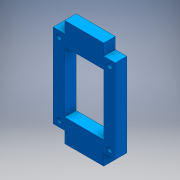
# Autodesk Inventor part: backFrame
Saved by Autodesk Inventor 2016 (Build 200138000, 138)
## iProperties
Created: 2016-06-05
Part Number: backFrame
Material: Generic
Document SubType Name: Modeling
Designer: hesaon
Density: 1 g/cm^3
Appearance: Default
Author: hesaon
Autodesk Inventor part; units mm, degrees
ref_plane "YZ Plane" through (0, 0, 0) normal (1, 0, 0) x (0, 1, 0)
ref_plane "XZ Plane" through (0, 0, 0) normal (0, 1, 0) x (-1, 0, 0)
ref_plane "XY Plane" through (0, 0, 0) normal (0, 0, 1) x (1, 0, 0)
sketch "Sketch1" plane through (0, 0, 0) normal (0, 1, 0) x (-1, 0, 0)
  line L0 (0, 0) -> (10, 0)
  line L1 (10, 0) -> (10, 10)
  line L2 (10, 10) -> (44, 10)
  line L3 (44, 10) -> (44, 0)
  line L4 (44, 0) -> (54, 0)
  line L5 (54, 0) -> (54, -73)
  line L6 (54, -73) -> (44, -73)
  line L7 (44, -73) -> (44, -83)
  line L8 (44, -83) -> (10, -83)
  line L9 (10, -83) -> (10, -73)
  line L10 (10, -73) -> (0, -73)
  line L11 (0, -73) -> (0, 0)
  dimension "d9" = 73
  dimension "d10" = 54
  dimension "thickness" = 10
  dimension "t" = 10
  dimension "d13" = 10
  dimension "d14" = 10
  dimension "d15" = 10
  dimension "d16" = 10
  dimension "d17" = 10
  constraints: 24 end point, 11 perpendicular, 1 coincident, 1 point on line, 1 vertical
  measures "d9" distance of L10.end point (0, 0)
  measures "d10" distance of point (0, 0) L4.end
  measures "thickness" distance of L0.end L1.end
  measures "t" distance of point (0, 0) L0.end
  measures "d13" distance of L3.end L4.end
  measures "d14" distance of L6.end L5.end
  measures "d15" distance of L8.end L9.end
  measures "d16" distance of L7.end L6.end
  measures "d17" distance from line of L11 L8.end
extrude "Extrusion1" add sketch "Sketch1" along normal blind 10
hole "Hole1" at (-49, 10, -5) direction (0, -1, 0) diameter 4.3 end through all
hole "Hole2" at (-5, 10, -5) direction (0, -1, 0) diameter 4.3 end through all
hole "Hole3" at (-5, 10, -68) direction (0, -1, 0) diameter 4.3 end through all
hole "Hole4" at (-49, 10, -68) direction (0, -1, 0) diameter 4.3 end through all
sketch "Sketch2" plane through (0, 10, 0) normal (0, 1, 0) x (1, 0, 0)
  circle A0 centre (-37, -5) radius 3.25
  circle A1 centre (-17, -5) radius 3.25
  circle A2 centre (-37, 78) radius 3.25
  circle A3 centre (-17, 78) radius 3.25
  line L0 (-44, -10) -> (-10, -10) projected
  line L1 (-10, 83) -> (-44, 83) projected
  line L2 (-44, 0) -> (-44, -10) projected
  line L3 (-10, -10) -> (-10, 0) projected
  line L4 (-10, 73) -> (-10, 83) projected
  line L5 (-44, 83) -> (-44, 73) projected
  point P0 (0, 0)
  dimension "d56" = 6.5
  dimension "d57" = 6.5
  dimension "d58" = 6.5
  dimension "d59" = 6.5
  dimension "d60" = 5
  dimension "d61" = 5
  dimension "d62" = 5
  dimension "d63" = 5
  dimension "d64" = 7
  dimension "d65" = 7
  dimension "d66" = 7
  dimension "d67" = 7
  constraints: 4 centre point
  measures "d56" diameter of A2
  measures "d57" diameter of A3
  measures "d58" diameter of A0
  measures "d59" diameter of A1
  measures "d60" distance from line of L0 A0.centre
  measures "d61" distance from line of L0 A1.centre
  measures "d62" distance from line of L1 A3.centre
  measures "d63" distance from line of L1 A2.centre
  measures "d64" distance from line of L2 A0.centre
  measures "d65" distance from line of L3 A1.centre
  measures "d66" distance from line of A3.centre L4
  measures "d67" distance from line of L5 A2.centre
extrude "Extrusion2" cut sketch "Sketch2" against normal blind 5
sketch "Sketch3" plane through (0, 0, 0) normal (0, -1, 0) x (1, 0, 0)
  line L0 (-44, -10) -> (-10, -10)
  line L1 (-10, -10) -> (-10, -63)
  line L2 (-10, -63) -> (-44, -63)
  line L3 (-44, -63) -> (-44, -10)
  line L4 (-10, 10) -> (-44, 10) projected
  line L5 (-44, -83) -> (-10, -83) projected
  line L6 (0, -73) -> (0, 0) projected
  line L7 (-54, 0) -> (-54, -73) projected
  dimension "d70" = 20
  dimension "d71" = 20
  dimension "d72" = 10
  dimension "d73" = 10
  constraints: 8 end point, 2 parallel, 1 horizontal, 1 perpendicular
  measures "d70" distance between parallel lines of L0 L4
  measures "d71" distance between parallel lines of L5 L2
  measures "d72" distance from line of L6 L0.end
  measures "d73" distance from line of L7 L0.start
extrude "Extrusion3" cut sketch "Sketch3" against normal blind 10
equation "\"thickness\" = t"
equation "\"d13\" = t"
equation "\"d14\" = t"
equation "\"d15\" = t"
equation "\"d16\" = t"
equation "\"d17\" = t"
equation "\"d18\" = t"
body "Solid1"
